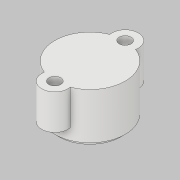
# Autodesk Inventor part: caster_body
Saved by Autodesk Inventor 2019.3 (Build 233278000, 278)
## iProperties
Created: 2019-03-11
Part Number: caster_body
Material: Generic
Document SubType Name: Modeling
Designer: Varga Daniel
Density: 1 g/cm^3
Appearance: White
Author: Varga Daniel
Autodesk Inventor part; units mm, degrees
ref_plane "YZ Plane" through (0, 0, 0) normal (1, 0, 0) x (0, 1, 0)
ref_plane "XZ Plane" through (0, 0, 0) normal (0, 1, 0) x (-1, 0, 0)
ref_plane "XY Plane" through (0, 0, 0) normal (0, 0, 1) x (1, 0, 0)
sketch "Sketch1" plane through (0, 0, 0) normal (0, 1, 0) x (-1, 0, 0)
  line L0 (0, 0) -> (23.6236, 0) construction
  line L1 (0, 0) -> (0, -20.0966) construction
  arc A0 (-8, 0) -> (8, 0) centre (0, 0) ccw
  arc A1 (-2.9468, -7.4375) -> (2.9468, -7.4375) centre (0, -8) ccw
  line L2 (0, -11) -> (-8.5189, -11) construction
  circle A2 centre (0, -8) radius 1.35
  line L3 (-8, 0) -> (8, 0)
  arc A3 (8, 0) -> (-8, 0) centre (0, 0) ccw
  arc A4 (2.9468, 7.4375) -> (-2.9468, 7.4375) centre (0, 8) ccw
  line L4 (0, 11) -> (-8.5189, 11) construction
  circle A5 centre (0, 8) radius 1.35
  dimension "d0" = 16
  dimension "d1" = 22
  dimension "d2" = 6
  dimension "d3" = 2.7
  constraints: 14 point on circle, 10 end point, 6 centre point, 6 symmetric about line, 3 coincident, 3 point on line, 1 collinear, 1 horizontal, 1 perpendicular, 1 tangent, 3 other
  measures "d0" diameter of A0
  measures "d1" diameter of L2 L0
  measures "d2" diameter of A1
  measures "d3" diameter of A2
extrude "Extrusion1" add sketch "Sketch1" along normal blind 8
extrude "Extrusion2" cut sketch "Sketch1" against normal blind 7 from surface at 8 contours A2 A0 | A0 A2 | A5 A3 | A3 A5
extrude "Extrusion3" add sketch "Sketch1" against normal blind 3.5 contours L3 A0 A2 | A3 A5 L3 | A2 A0 | A3 A5 picked at (0, -7.5415) picked at (0, 7.5415)
chamfer "Chamfer1" distance 1 angle 45 1 edges at (2.9468, -3.5, 7.4375)
body "Solid1"
